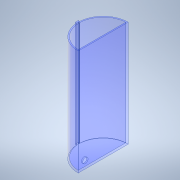
# Autodesk Inventor part: Deposito_Líquido
Saved by Autodesk Inventor 2020 (Build 240168000, 168)
## iProperties
Created: 2020-10-28
Part Number: Deposito_Líquido
Material: PET Plastic
Document SubType Name: Modeling
Designer: aaron
Density: 1.541 g/cm^3
Appearance: Clear - Blue
Author: aaron
Autodesk Inventor part; units mm, degrees
ref_plane "YZ Plane" through (0, 0, 0) normal (1, 0, 0) x (0, 1, 0)
ref_plane "XZ Plane" through (0, 0, 0) normal (0, 1, 0) x (-1, 0, 0)
ref_plane "XY Plane" through (0, 0, 0) normal (0, 0, 1) x (1, 0, 0)
sketch "Sketch1" plane through (0, 0, 0) normal (0, 1, 0) x (-1, 0, 0)
  arc A0 (41.4246, 2.5) -> (41.4246, -2.5) centre (0, 0) ccw construction
  line L0 (0, -41.5) -> (0, 41.5)
  line L1 (0, 0) -> (41.5, 0) construction
  line L2 (41.4246, 2.5) -> (43.7, 2.5)
  line L3 (43.7, 2.5) -> (43.7, -2.5)
  line L4 (43.7, -2.5) -> (41.4246, -2.5)
  line L5 (39.3, 2.5) -> (43.7, -2.5) construction
  line L6 (43.7, 2.5) -> (39.3, -2.5) construction
  arc A1 (0, -41.5) -> (41.4246, -2.5) centre (0, 0) ccw
  arc A2 (41.4246, 2.5) -> (0, 41.5) centre (0, 0) ccw
  line L7 (41.4246, -2.5) -> (41.4246, 2.5) construction
  line L8 (2, 39.4493) -> (2, -39.4493)
  arc A3 (2, -39.4493) -> (39.4968, -0.5) centre (0, 0) ccw
  line L9 (39.4968, -0.5) -> (41.7, -0.5)
  line L10 (41.7, -0.5) -> (41.7, 0.5)
  line L11 (41.7, 0.5) -> (39.4968, 0.5)
  arc A4 (39.4968, 0.5) -> (2, 39.4493) centre (0, 0) ccw
  dimension "d0" = 83
  dimension "d1" = 83
  dimension "d2" = 5
  dimension "d4" = 2.2
  dimension "d5" = 41.5
  dimension "d6" = 2
  constraints: 24 end point, 12 point on circle, 5 centre point, 2 midpoint, 2 parallel, 2 perpendicular, 2 vertical, 1 coincident, 1 horizontal, 5 other
  measures "d0" diameter of A0
  measures "d1" distance of L0.start L0.end
  measures "d2" distance of L2.end L3.end
  measures "d4" distance from line of L3 L1.end
  measures "d5" distance of point (0, 0) L1.end
  measures "d6" distance between parallel lines of L0 L8
extrude "Extrusion1" add sketch "Sketch1" against normal blind 2 contours L0 A2 L2 L3 L4 A1 | A4 L11 L10 L9 A3 L8
extrude "Extrusion2" add sketch "Sketch1" along normal blind 173
sketch "Sketch2" plane through (0, -2, 41.5) normal (1, 0, 0) x (0, 0, -1)
  circle A0 centre (12, 12) radius 4.5
  line L0 (83, 0) -> (0, 0) projected
  line L1 (0, 0) -> (0, 175) projected
  point P0 (41.5, 2)
  dimension "d11" = 9
  dimension "d12" = 12
  dimension "d13" = 12
  constraints: 1 centre point
  measures "d11" diameter of A0
  measures "d12" distance from line of L0 A0.centre
  measures "d13" distance from line of L1 A0.centre
extrude "Extrusion3" cut sketch "Sketch2" against normal blind 10
body "Solid1"
